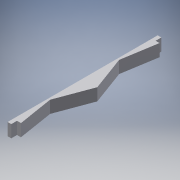
# Autodesk Inventor part: short_insert_invert_CPY1
Saved by Autodesk Inventor 2017 (Build 210142000, 142)
## iProperties
Created: 2018-01-15
Part Number: short_insert_invert_CPY1
Material: Generic
Document SubType Name: Modeling
Designer: Mitch
Density: 1 g/cm^3
Appearance: White
Author: Mitch
Autodesk Inventor part; units mm, degrees
ref_plane "YZ Plane" through (0, 0, 0) normal (1, 0, 0) x (0, 1, 0)
ref_plane "XZ Plane" through (0, 0, 0) normal (0, 1, 0) x (-1, 0, 0)
ref_plane "XY Plane" through (0, 0, 0) normal (0, 0, 1) x (1, 0, 0)
sketch "Sketch1" plane through (0, 0, 0) normal (0, 1, 0) x (-1, 0, 0)
  line L0 (0, 0) -> (0, -61.8744)
  line L1 (0, 0) -> (-3.4036, 0)
  line L2 (0, -61.8744) -> (-3.4036, -61.8744)
  line L3 (-3.4036, 0) -> (-0.889, -15.5448)
  line L4 (-0.889, -15.5448) -> (-6.5786, -30.9015)
  line L5 (-6.5786, -30.9015) -> (-0.889, -46.3296)
  line L6 (-0.889, -46.3296) -> (-3.4036, -61.8744)
  dimension "d0" = 61.8744
  dimension "d1" = 3.4036
  dimension "d2" = 3.4036
  dimension "d3" = 15.5448
  dimension "d4" = 31.0642
  dimension "d5" = 15.5448
  dimension "d6" = 0.889
  dimension "d7" = 0.889
  dimension "d10" = 6.5786
  constraints: 14 end point, 2 horizontal, 1 vertical
  measures "d0" distance of L0.start L0.end
  measures "d1" distance of L0.start L1.end
  measures "d2" distance of L0.end L2.end
  measures "d3" vertical distance of L3.end L1.end
  measures "d4" distance of L4.end L1.end
  measures "d5" vertical distance of L5.end L2.end
  measures "d6" distance from line of L3.end L0
  measures "d7" distance from line of L0 L5.end
  measures "d10" distance from line of L0 L4.end
extrude "Extrusion1" add sketch "Sketch1" along normal blind 7.3025
sketch "Sketch2" plane through (0, 0, 0) normal (0, 0, 1) x (1, 0, 0)
  line L0 (3.4036, 0) -> (0, 0) projected
  line L1 (1.651, 0) -> (0, 0)
  line L2 (0, 7.3025) -> (1.651, 7.3025)
  line L3 (1.651, 7.3025) -> (1.651, 0)
  line L4 (1.651, 0) -> (0, 0)
  line L5 (0, 0) -> (0, 7.3025)
  dimension "d17" = 1.651
  constraints: 10 end point, 2 parallel, 1 horizontal, 1 perpendicular, 1 point on line
  measures "d17" distance between parallel lines of L3 L5
sketch "Sketch3" plane through (3.4036, 0, -61.8744) normal (0, 0, -1) x (-1, 0, 0)
  line L0 (3.4036, 7.3025) -> (0, 7.3025) projected
  line L1 (0, 0) -> (3.4036, 0) projected
  line L2 (3.4036, 7.3025) -> (1.7526, 7.3025)
  line L3 (1.7526, 7.3025) -> (1.7526, 0)
  line L4 (1.7526, 0) -> (3.4036, 0)
  line L5 (3.4036, 0) -> (3.4036, 7.3025)
  dimension "d12" = 1.651
  constraints: 8 end point, 2 parallel, 1 horizontal, 1 perpendicular, 1 point on line
  measures "d12" distance of L4.end L3.end
extrude "Extrusion2" add sketch "Sketch3" along normal blind 2.5654
extrude "Extrusion3" add sketch "Sketch2" along normal blind 2.5654
body "Solid1"
